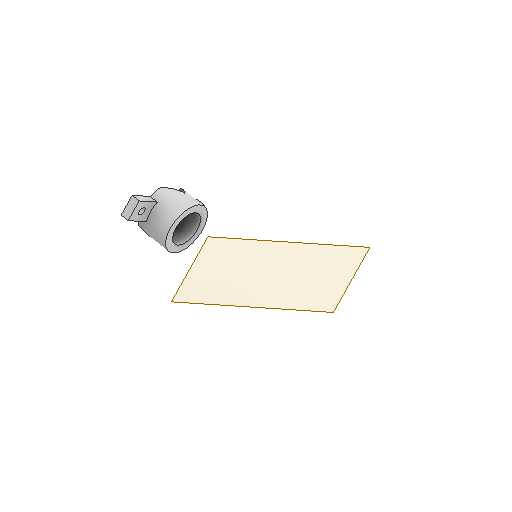
# Autodesk Inventor part: Condenser_holder_frame
Saved by Autodesk Inventor 2023 (Build 270158000, 158)
## iProperties
Created: 2021-08-11
Part Number: Condenser_holder_frame
Material: Generic
Document SubType Name: Modeling
Designer: CDT
Density: 1 g/cm^3
Appearance: Default
Author: CDT
Autodesk Inventor part; units mm, degrees
ref_plane "YZ Plane" through (0, 0, 0) normal (1, 0, 0) x (0, 1, 0)
ref_plane "XZ Plane" through (0, 0, 0) normal (0, 1, 0) x (-1, 0, 0)
ref_plane "XY Plane" through (0, 0, 0) normal (0, 0, 1) x (1, 0, 0)
ref_plane "Work Plane1" through (-1.5995, -66.1757, -63.553) normal (0.9860009, -0.1658848, 0.0168677) x (-0.1508814, -0.8445852, 0.5137224)
sketch "Sketch1" plane through (-1.5995, -66.1757, -63.553) normal (0.9860009, -0.1658848, 0.0168677) x (-0.1508814, -0.8445852, 0.5137224)
  line L0 (-19.4838, -68.3172) -> (-27.4838, -68.3172)
  line L1 (-27.4838, -68.3172) -> (-27.4838, -108.3172)
  line L2 (-27.4838, -108.3172) -> (-19.4838, -108.3172)
  line L3 (-19.4838, -108.3172) -> (-19.4838, -68.3172)
  circle A0 centre (-23.4838, -88.3172) radius 9.75
  circle A1 centre (-23.4838, -73.3172) radius 1.5
  circle A2 centre (-23.4838, -103.3172) radius 1.5
  point P0 (-27.4838, -79.4254)
  point P1 (-27.4838, -97.2089)
  point P2 (-19.4838, -97.2089)
  point P3 (-19.4838, -79.4254)
  dimension "d0" = 19.5
  dimension "d1" = 4
  dimension "d2" = 4
  dimension "d3" = 20
  dimension "d4" = 20
  dimension "d5" = 3
  dimension "d6" = 3
  dimension "d8" = 15
  dimension "d9" = 15
  constraints: 8 end point, 3 centre point, 2 parallel, 1 coincident, 1 horizontal, 1 perpendicular
  measures "d0" diameter of A0
  measures "d1" distance from line of L3 point (-23.484, -88.317)
  measures "d2" distance from line of L1 point (-23.484, -88.317)
  measures "d3" distance from line of L2 point (-23.484, -88.317)
  measures "d4" distance from line of L0 point (-23.484, -88.317)
  measures "d5" diameter of A1
  measures "d6" diameter of A2
  measures "d8" distance of point (-23.484, -88.317) A2.centre
  measures "d9" distance of A1.centre point (-23.484, -88.317)
extrude "Extrusion1" add sketch "Sketch1" along normal blind 3.5
sketch "Sketch2" plane through (1.8515, -66.7563, -63.494) normal (0.9860009, -0.1658848, 0.0168677) x (-0.1508814, -0.8445852, 0.5137224)
  circle A0 centre (-23.4838, -88.3172) radius 9.75
  dimension "d32" = 19.5
  constraints: 1 centre point, 1 coincident
  measures "d32" diameter of A0
extrude "Extrusion2" add sketch "Sketch2" along normal blind 10
ref_plane "Work Plane2" through (-12, -44.9283, 0) normal (0, 0, 1) x (1, 0, 0)
sketch "Sketch3" plane through (21.5228, -3.621, 0.3682) normal (0.9860009, -0.1658848, 0.0168677) x (0.0171047, 0, -0.9998537)
  circle A0 centre (0, 0) radius 6.55
  point P0 (0, 0)
  dimension "d14" = 13.1
  constraints: 1 centre point, 1 coincident
  measures "d14" diameter of A0
extrude "Extrusion3" cut sketch "Sketch3" against normal up to surface (13.5 mm away)
sketch "Sketch5" plane through (-1.5995, -66.1757, -63.553) normal (-0.9860009, 0.1658848, -0.0168677) x (-0.1508814, -0.8445852, 0.5137224)
  line L0 (-11.4838, 94.3172) -> (-35.4838, 94.3172)
  line L1 (-35.4838, 94.3172) -> (-35.4838, 82.3172)
  line L2 (-35.4838, 82.3172) -> (-11.4838, 82.3172)
  line L3 (-11.4838, 82.3172) -> (-11.4838, 94.3172)
  line L4 (-27.4838, 108.3172) -> (-19.4838, 108.3172) projected
  line L5 (-19.4838, 68.3172) -> (-27.4838, 68.3172) projected
  point P0 (-23.4838, 88.3172)
  dimension "d36" = 14
  dimension "d37" = 14
  dimension "d38" = 12
  dimension "d39" = 12
  dimension "d54" = 12
  constraints: 8 end point, 2 parallel, 1 horizontal, 1 perpendicular
  measures "d36" distance between parallel lines of L4 L0
  measures "d37" distance between parallel lines of L5 L2
  measures "d38" distance from line of L3 point (-23.484, 88.317)
  measures "d39" distance from line of L1 point (-23.484, 88.317)
  measures "d54" distance between parallel lines of L2 L0
extrude "Extrusion5" cut sketch "Sketch5" against normal blind 6
chamfer "Chamfer6" [suppressed]
chamfer "Chamfer7" distance 6 angle 45 4 edges at (15.3336, 5.0321, 2.7396) (13.7777, -3.6776, 8.0373) (12.926, -9.7865, -2.2561) (14.4819, -1.0768, -7.5539)
equation "\"d2\" = d1"
equation "\"d37\" = d36"
equation "\"d39\" = d38"
body "Solid1"
